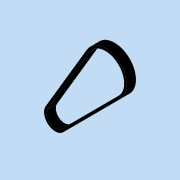
# Autodesk Inventor part: Pas zębaty 10 T5-295
Saved by Autodesk Inventor 2018 (Build 220112000, 112)
## iProperties
Created: 2019-02-09
Part Number: Pas zębaty 10 T5-295
Material: Ogólny
Document SubType Name: Modeling
Designer: Dawid
Density: 1 g/cm^3
Appearance: Anodowana - czarna
Author: Dawid
Autodesk Inventor part; units mm, degrees
ref_plane "YZ Plane" through (0, 0, 0) normal (1, 0, 0) x (0, 1, 0)
ref_plane "XZ Plane" through (0, 0, 0) normal (0, 1, 0) x (-1, 0, 0)
ref_plane "XY Plane" through (0, 0, 0) normal (0, 0, 1) x (1, 0, 0)
sketch "Szkic1" plane through (0, 0, 0) normal (0, 1, 0) x (-1, 0, 0)
  arc A0 (48.2455, -77.7225) -> (63.1896, -66.1474) centre (54.9934, -71) ccw
  arc A1 (46.3327, -79.628) -> (65.5129, -64.7719) centre (54.9934, -71) ccw
  arc A2 (17.7907, 10.5331) -> (-14.647, -14.5918) centre (0, 0) ccw
  arc A3 (20.1141, 11.9086) -> (-16.5598, -16.4974) centre (0, 0) ccw
  line L0 (65.5129, -64.7719) -> (20.1141, 11.9086)
  line L1 (46.3327, -79.628) -> (-16.5598, -16.4974)
  line L2 (17.7907, 10.5331) -> (63.1896, -66.1474)
  line L3 (48.2455, -77.7225) -> (-14.647, -14.5918)
  point P0 (0, 0)
  constraints: 8 end point, 8 point on circle, 8 tangent, 4 centre point, 2 coincident, 4 other
extrude "Wyciągnięcie proste1" add sketch "Szkic1" along normal blind 10
